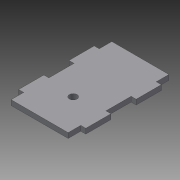
# Autodesk Inventor part: bottom
Saved by Autodesk Inventor 2015 (Build 190159000, 159)
## iProperties
Created: 2017-03-04
Part Number: bottom
Material: Generic
Document SubType Name: Modeling
Designer: Guy
Density: 1 g/cm^3
Appearance: Default
Author: Guy
Autodesk Inventor part; units mm, degrees
ref_plane "YZ Plane" through (0, 0, 0) normal (1, 0, 0) x (0, 1, 0)
ref_plane "XZ Plane" through (0, 0, 0) normal (0, 1, 0) x (-1, 0, 0)
ref_plane "XY Plane" through (0, 0, 0) normal (0, 0, 1) x (1, 0, 0)
sketch "Sketch1" plane through (0, 0, 0) normal (0, 0, 1) x (1, 0, 0)
  line L0 (0, 0) -> (120, 0)
  line L1 (120, 0) -> (120, 80)
  line L2 (120, 80) -> (0, 80)
  line L3 (0, 80) -> (0, 0)
  dimension "d0" = 120
  dimension "d1" = 80
  constraints: 8 end point, 2 parallel, 1 horizontal, 1 perpendicular
  measures "d0" distance of L2.end L1.end
  measures "d1" distance of L0.end L1.end
extrude "Extrusion1" add sketch "Sketch1" along normal blind 6
sketch "Sketch2" plane through (0, 0, 6) normal (0, 0, 1) x (1, 0, 0)
  line L0 (0, 0) -> (120, 0) projected
  line L1 (120, 0) -> (120, 80) projected
  line L2 (120, 80) -> (0, 80) projected
  line L3 (0, 80) -> (0, 0) projected
  line L4 (120, 0) -> (105, 0)
  line L5 (105, 0) -> (105, 6)
  line L6 (105, 6) -> (120, 6)
  line L7 (120, 6) -> (120, 0)
  line L8 (0, 0) -> (120, 0) projected
  line L9 (75, 0) -> (45, 0)
  line L10 (45, 0) -> (45, 6)
  line L11 (45, 6) -> (75, 6)
  line L12 (75, 6) -> (75, 0)
  line L13 (15, 0) -> (0, 0)
  line L14 (0, 0) -> (0, 6)
  line L15 (0, 6) -> (15, 6)
  line L16 (15, 6) -> (15, 0)
  line L17 (120, 80) -> (105, 80)
  line L18 (105, 80) -> (105, 74)
  line L19 (105, 74) -> (120, 74)
  line L20 (120, 74) -> (120, 80)
  line L21 (120, 80) -> (0, 80) projected
  line L22 (75, 80) -> (45, 80)
  line L23 (45, 80) -> (45, 74)
  line L24 (45, 74) -> (75, 74)
  line L25 (75, 74) -> (75, 80)
  line L26 (15, 80) -> (0, 80)
  line L27 (0, 80) -> (0, 74)
  line L28 (0, 74) -> (15, 74)
  line L29 (15, 74) -> (15, 80)
  dimension "d4" = 6
  dimension "d5" = 6
  dimension "d6" = 15
  dimension "d7" = 15
  dimension "d8" = 30
  dimension "d10" = 30
  constraints: 48 end point, 12 parallel, 10 point on line, 6 horizontal, 6 perpendicular, 4 collinear
  measures "d4" distance between parallel lines of L6 L4
  measures "d5" distance between parallel lines of L26 L28
  measures "d6" distance between parallel lines of L5 L1
  measures "d7" distance between parallel lines of L16 L14
  measures "d8" distance between parallel lines of L12 L10
  measures "d10" distance between parallel lines of L5 L12
extrude "Extrusion2" cut sketch "Sketch2" against normal up to next contours L3 L15 L16 L0 | L10 L11 L12 L0 | L3 L2 L29 L28 | L5 L6 L1 L0 | L2 L25 L24 L23 | L19 L18 L2 L1
sketch "Sketch3" plane through (0, 0, 6) normal (0, 0, 1) x (1, 0, 0)
  circle A0 centre (80, 40) radius 4.6
  line L0 (75, 0) -> (105, 0) projected
  line L1 (120, 6) -> (120, 74) projected
  point P0 (0, 0)
  dimension "d13" = 9.2
  dimension "d14" = 40
  dimension "d15" = 40
  constraints: 1 centre point
  measures "d13" diameter of A0
  measures "d14" distance from line of A0.centre L0
  measures "d15" distance from line of L1 A0.centre
extrude "Extrusion3" cut sketch "Sketch3" against normal up to next
body "Solid1"
